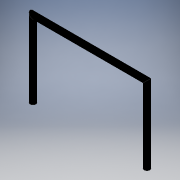
# Autodesk Inventor part: Leg
Saved by Autodesk Inventor 2016 (Build 200138000, 138)
## iProperties
Created: 2017-12-15
Part Number: Leg
Material: Generic
Document SubType Name: Modeling
Designer: sun01147
Density: 1 g/cm^3
Appearance: Default
Author: sun01147
Autodesk Inventor part; units mm, degrees
ref_plane "YZ Plane" through (0, 0, 0) normal (1, 0, 0) x (0, 1, 0)
ref_plane "XZ Plane" through (0, 0, 0) normal (0, 1, 0) x (-1, 0, 0)
ref_plane "XY Plane" through (0, 0, 0) normal (0, 0, 1) x (1, 0, 0)
sketch "Sketch1" plane through (0, 0, 0) normal (0, 0, 1) x (1, 0, 0)
  line L0 (0, 10.16) -> (0, 0)
  line L1 (0, 10.16) -> (15.24, 10.16)
  line L2 (15.24, 10.16) -> (15.24, 0)
  dimension "d0" = 10.16
  dimension "d4" = 15.24
  dimension "d7" = 10.16
  constraints: 6 end point, 2 vertical, 1 horizontal
  measures "d0" distance of L0.start L0.end
  measures "d4" distance of L0.start L1.end
  measures "d7" distance of L1.end L2.end
sketch "Sketch3" plane through (0, 0, 0) normal (0, 1, 0) x (-1, 0, 0)
  circle A0 centre (0, 0) radius 0.381
  circle A1 centre (-15.2457, 0) radius 0.381
  dimension "d5" = 0.762
  dimension "d6" = 0.762
  constraints: 2 centre point, 1 coincident
  measures "d5" diameter of A0
  measures "d6" diameter of A1
sweep "Sweep1" add profiles "Sketch3" path "Sketch1" contours A0
body "Solid1"
